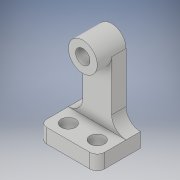
# Autodesk Inventor part: Part1
Saved by Autodesk Inventor 2018 (Build 220112000, 112)
## iProperties
Created: 2019-01-23
Part Number: Part1
Material: Generic
Document SubType Name: Modeling
Designer: russd
Density: 1 g/cm^3
Appearance: Default
Author: russd
Autodesk Inventor part; units mm, degrees
ref_plane "YZ Plane" through (0, 0, 0) normal (1, 0, 0) x (0, 1, 0)
ref_plane "XZ Plane" through (0, 0, 0) normal (0, 1, 0) x (-1, 0, 0)
ref_plane "XY Plane" through (0, 0, 0) normal (0, 0, 1) x (1, 0, 0)
sketch "Sketch1" plane through (0, 0, 0) normal (0, 0, 1) x (1, 0, 0)
  line L0 (-3.9739, 11.3944) -> (46.8261, 11.3944)
  line L1 (46.8261, 11.3944) -> (46.8261, -71.1556)
  line L2 (46.8261, -71.1556) -> (-3.9739, -71.1556)
  line L3 (-3.9739, -71.1556) -> (-3.9739, 11.3944)
  point P0 (0, 0)
  dimension "d0" = 50.8
  dimension "d1" = 82.55
  constraints: 8 end point, 2 parallel, 1 horizontal, 1 perpendicular
  measures "d0" distance of L1.end L2.end
  measures "d1" distance of L0.end L1.end
extrude "Extrusion1" add sketch "Sketch1" along normal blind 38.1
sketch "Sketch2" plane through (46.8261, -71.1556, 0) normal (1, 0, 0) x (0, 0, -1)
  line L0 (0, 82.55) -> (-38.1, 82.55) projected
  line L1 (-38.1, 82.55) -> (-12.7, 82.55)
  line L2 (-12.7, 82.55) -> (-12.7, 12.7)
  line L3 (-12.7, 12.7) -> (-38.1, 12.7)
  line L4 (-38.1, 12.7) -> (-38.1, 82.55)
  point P0 (0, 71.1556)
  dimension "d4" = 25.4
  dimension "d5" = 69.85
  constraints: 8 end point, 2 parallel, 1 horizontal, 1 perpendicular
  measures "d4" distance of L2.end L3.end
  measures "d5" distance of L1.end L2.end
extrude "Extrusion2" cut sketch "Sketch2" against normal through all
sketch "Sketch3" plane through (46.8261, -58.4556, 12.7) normal (0, 0, 1) x (1, 0, 0)
  line L0 (-50.8, 69.85) -> (0, 69.85) projected
  line L1 (-50.8, 69.85) -> (-38.1, 69.85)
  line L2 (-38.1, 69.85) -> (-38.1, 0)
  line L3 (-38.1, 0) -> (-50.8, 0)
  line L4 (-50.8, 0) -> (-50.8, 69.85)
  line L5 (0, 69.85) -> (-12.7, 69.85)
  line L6 (-12.7, 69.85) -> (-12.7, 0)
  line L7 (-12.7, 0) -> (0, 0)
  line L8 (0, 0) -> (0, 69.85)
  point P0 (-46.8261, 58.4556)
  dimension "d8" = 12.7
  dimension "d9" = 69.85
  dimension "d10" = 12.7
  dimension "d11" = 69.85
  constraints: 16 end point, 4 parallel, 2 horizontal, 2 perpendicular
  measures "d8" distance of L2.end L3.end
  measures "d9" distance of L1.end L2.end
  measures "d10" distance of L7.end L6.end
  measures "d11" distance of L6.end L5.end
extrude "Extrusion3" cut sketch "Sketch3" against normal through all
sketch "Sketch4" plane through (8.7261, -58.4556, 12.7) normal (0, 0, 1) x (1, 0, 0)
  line L0 (0, 69.85) -> (0, 0) construction
  line L1 (25.4, 0) -> (0, 0) construction
  line L2 (25.4, 0) -> (25.4, 69.85) construction
  line L3 (0, 69.85) -> (25.4, 69.85) construction
  circle A0 centre (12.7, 57.15) radius 12.7
  circle A1 centre (12.7, 57.15) radius 6.35
  point P0 (-8.7261, 58.4556)
  dimension "d14" = 12.7
  constraints: 3 tangent, 2 centre point, 1 coincident
  measures "d14" diameter of A1
extrude "Extrusion4" add sketch "Sketch4" along normal mid plane 25.4
sketch "Sketch5" plane through (8.7261, 11.3944, 12.7) normal (0, 0, 1) x (1, 0, 0)
  arc A0 (12.7, 0) -> (0, -12.7) centre (12.7, -12.7) ccw projected
  line L0 (0, 0) -> (12.7, 0) projected
  line L1 (0, 0) -> (0, -12.7) projected
  arc A1 (25.4, -12.7) -> (12.7, 0) centre (12.7, -12.7) ccw projected
  line L2 (25.4, -12.7) -> (25.4, 0) projected
  line L3 (12.7, 0) -> (25.4, 0) projected
  point P0 (-8.7261, -11.3944)
extrude "Extrusion5" cut sketch "Sketch5" against normal through all
sketch "Sketch6" plane through (21.4261, -1.3056, 12.7) normal (0, 0, 1) x (1, 0, 0)
  circle A0 centre (0, 0) radius 6.35 projected
  point P0 (-21.4261, 1.3056)
extrude "Extrusion6" cut sketch "Sketch6" against normal through all
sketch "Sketch7" plane through (46.8261, -58.4556, 38.1) normal (0, 1, 0) x (1, 0, 0)
  line L0 (-50.8, 0) -> (-50.8, 38.1) construction
  line L1 (0, 0) -> (-50.8, 0) construction
  line L2 (0, 38.1) -> (0, 0) construction
  line L3 (-12.7, 38.1) -> (0, 38.1) construction
  line L4 (-12.7, 25.4) -> (-12.7, 38.1) construction
  line L5 (-12.7, 25.4) -> (-38.1, 25.4) construction
  line L6 (-38.1, 25.4) -> (-38.1, 38.1) construction
  line L7 (-50.8, 38.1) -> (-38.1, 38.1) construction
  line L8 (-50.8, 0) -> (-50.8, 38.1) construction
  line L9 (0, 0) -> (-50.8, 0) construction
  line L10 (0, 38.1) -> (0, 0) construction
  line L11 (-12.7, 38.1) -> (0, 38.1) construction
  line L12 (-12.7, 25.4) -> (-12.7, 38.1) construction
  line L13 (-12.7, 25.4) -> (-38.1, 25.4) construction
  line L14 (-38.1, 25.4) -> (-38.1, 38.1) construction
  line L15 (-50.8, 38.1) -> (-38.1, 38.1) construction
  line L16 (-38.1, 12.7) -> (-12.7, 12.7) construction
  point P0 (-46.8261, 38.1)
  constraints: 2 coincident
hole "Hole1" at (8.7261, -58.4556, 25.4) at (34.1261, -58.4556, 25.4) direction (0, -1, 0) diameter 12.7 end through all
fillet "Fillet1" radius 6.35 2 edges at (-3.9739, -64.8056, 38.1) (46.8261, -64.8056, 38.1)
fillet "Fillet2" radius 12.7 2 edges at (8.7261, -58.4556, 6.35) (34.1261, -58.4556, 6.35)
body "Solid1"
